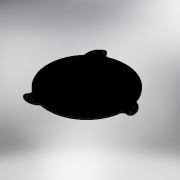
# Autodesk Inventor part: Plateau metalique
Saved by Autodesk Inventor 2017 (Build 210142000, 142)
## iProperties
Company: FABLAB Frenchmakers
Part Number: Plateau metalique
Project: 1420 VAUBAN 3D XL
Material: Aluminium
Catalog Web Link: http://www.frenchmakers.com/
Document SubType Name: Modeling
Designer: FABLAB Frenchmakers
Mass: 268.373 g
Surface Area: 685.958 cm^2
Volume: 99.3976 cm^3
Density: 2.7 g/cm^3
Appearance: Anodisé - Noir
Stock Number: 1420-04-01
Autodesk Inventor part; units mm, degrees
ref_plane "YZ Plane" through (0, 0, 0) normal (1, 0, 0) x (0, 1, 0)
ref_plane "XZ Plane" through (0, 0, 0) normal (0, 1, 0) x (-1, 0, 0)
ref_plane "XY Plane" through (0, 0, 0) normal (0, 0, 1) x (1, 0, 0)
sketch "Esquisse2" plane through (0, 0, 0) normal (0, 0, 1) x (1, 0, 0)
  circle A0 centre (0, 0) radius 100
  dimension "Diamètre" = 200
  constraints: 1 centre point, 1 coincident
  measures "Diamètre" diameter of A0
extrude "Embase" add sketch "Esquisse2" against normal blind 3
sketch "Esquisse1" plane through (0, 0, 0) normal (0, 0, 1) x (1, 0, 0)
  arc A0 (99.7184, -7.5) -> (95.3938, 30.0004) centre (0, 0) ccw
  arc A1 (119.4999, -0.1943) -> (95.3938, 30.0004) centre (89.51, 0.583) ccw
  line L0 (99.7184, -7.5) -> (112.0024, -7.5)
  arc A2 (112.0024, -7.5) -> (119.4999, -0.1943) centre (112.0024, 0) ccw
  point P0 (106.4504, 15)
  point P1 (106.4504, 15)
  dimension "d0" = 200
  dimension "d1" = 60
  dimension "d2" = 89.51
  dimension "d3" = 0.583
  dimension "d4" = 7.5
  dimension "d5" = 15
  dimension "d9" = 15
  dimension "d10" = 5.552
  constraints: 6 point on circle, 3 centre point, 2 coincident, 2 end point, 2 tangent, 1 horizontal
  measures "d0" diameter of A0
  measures "d1" diameter of A1
  measures "d2" horizontal distance of point (0, 0) A1.centre
  measures "d3" vertical distance of point (0, 0) A1.centre
  measures "d4" distance from line of point (0, 0) L0
  measures "d5" diameter of A2
  measures "d9" vertical distance of A2.centre point (106.45, 15)
  measures "d10" horizontal distance of A2.centre point (106.45, 15)
extrude "Oreille" add sketch "Esquisse1" against normal up to surface (3 mm away)
hole "M3" at (106.4504, 15, 0) direction (0, 0, -1) diameter 2.459 depth 8.8 tip angle 118 thread size "M3x0.5" class "6H" standard "ISO Metric profile"
hole "Passage vis" at (112.0024, 0, 0) direction (0, 0, -1) diameter 5.5 end through all
fillet "Congé1" radius 8 2 edges at (99.7184, -7.5, -1.5) (95.3938, 30.0004, -1.5)
pattern_circular "Réseau circulaire1" count 3 over 360 about axis through (0, 0, -10) along (0, 0, 1) of "Congé1", "Passage vis", "M3", "Oreille"
equation "\"d0\" = Diamètre"
